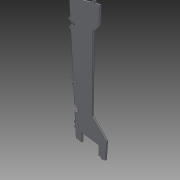
# Autodesk Inventor part: inner_brace_left
Saved by Autodesk Inventor 2014 (Build 180170000, 170)
## iProperties
Created: 2014-04-02
Part Number: inner_brace_left
Material: Plywood, Finish
Document SubType Name: Modeling
Designer: buben
Density: 0.552 g/cm^3
Appearance: Plywood - New
Author: buben
Autodesk Inventor part; units mm, degrees
ref_plane "YZ Plane" through (0, 0, 0) normal (1, 0, 0) x (0, 1, 0)
ref_plane "XZ Plane" through (0, 0, 0) normal (0, 1, 0) x (-1, 0, 0)
ref_plane "XY Plane" through (0, 0, 0) normal (0, 0, 1) x (1, 0, 0)
sketch "Sketch1" plane through (0, 0, 0) normal (0, 1, 0) x (-1, 0, 0)
  line L0 (0, 0) -> (0, -489)
  line L1 (0, -489) -> (-30.25, -489)
  line L2 (-30.25, -489) -> (-30.25, -439)
  line L3 (-30.25, -439) -> (-112.25, -439)
  line L4 (-112.25, -439) -> (-112.25, -489)
  line L5 (-112.25, -489) -> (-142.5, -489)
  line L6 (-142.5, -489) -> (-142.5, -399)
  line L7 (-142.5, -399) -> (-80, -336.5)
  line L8 (-80, -336.5) -> (-80, -65)
  line L9 (-80, -65) -> (-100, -45)
  line L10 (-100, -45) -> (-100, 0)
  line L11 (-100, 0) -> (0, 0)
  dimension "d0" = 135
  dimension "d1" = 100
  dimension "d2" = 489
  dimension "d3" = 45
  dimension "d4" = 20
  dimension "d5" = 30.25
  dimension "d6" = 50
  dimension "d7" = 82
  dimension "d8" = 40
  constraints: 24 end point, 7 parallel, 3 collinear, 2 perpendicular, 1 vertical
  measures "d0" angle of L9 L10
  measures "d1" distance of L10.end L0.start
  measures "d2" distance of L0.start L0.end
  measures "d3" distance of L9.end L10.end
  measures "d4" horizontal distance of L8.end L9.end
  measures "d5" distance of L0.end L1.end
  measures "d6" distance of L1.end L2.end
  measures "d7" distance of L2.end L3.end
  measures "d8" vertical distance of L6.end L3.end
extrude "Extrusion1" add sketch "Sketch1" along normal blind 6.5
sketch "Sketch2" plane through (0, 6.5, 0) normal (0, 1, 0) x (1, 0, 0)
  line L0 (0, 0) -> (100, 0) projected
  line L1 (30.25, 489) -> (0, 489) projected
  line L2 (0, 489) -> (0, 0) projected
  line L3 (16.3, 425.75) -> (16.3, 421.25)
  line L4 (0, 421.25) -> (0, 425.75)
  line L5 (5, 428.25) -> (12.3, 428.25)
  line L6 (12.3, 418.75) -> (5, 418.75)
  line L7 (0, 425.75) -> (5, 425.75)
  line L8 (12.3, 425.75) -> (16.3, 425.75)
  line L9 (16.3, 421.25) -> (12.3, 421.25)
  line L10 (5, 421.25) -> (0, 421.25)
  line L11 (5, 418.75) -> (5, 421.25)
  line L12 (5, 425.75) -> (5, 428.25)
  line L13 (12.3, 428.25) -> (12.3, 425.75)
  line L14 (12.3, 421.25) -> (12.3, 418.75)
  line L15 (16.3, 246.75) -> (16.3, 242.25)
  line L16 (0, 242.25) -> (0, 246.75)
  line L17 (5, 249.25) -> (12.3, 249.25)
  line L18 (12.3, 239.75) -> (5, 239.75)
  line L19 (0, 246.75) -> (5, 246.75)
  line L20 (12.3, 246.75) -> (16.3, 246.75)
  line L21 (16.3, 242.25) -> (12.3, 242.25)
  line L22 (5, 242.25) -> (0, 242.25)
  line L23 (5, 239.75) -> (5, 242.25)
  line L24 (5, 246.75) -> (5, 249.25)
  line L25 (12.3, 249.25) -> (12.3, 246.75)
  line L26 (12.3, 242.25) -> (12.3, 239.75)
  line L27 (16.3, 67.75) -> (16.3, 63.25)
  line L28 (0, 63.25) -> (0, 67.75)
  line L29 (5, 70.25) -> (12.3, 70.25)
  line L30 (12.3, 60.75) -> (5, 60.75)
  line L31 (0, 67.75) -> (5, 67.75)
  line L32 (12.3, 67.75) -> (16.3, 67.75)
  line L33 (16.3, 63.25) -> (12.3, 63.25)
  line L34 (5, 63.25) -> (0, 63.25)
  line L35 (5, 60.75) -> (5, 63.25)
  line L36 (5, 67.75) -> (5, 70.25)
  line L37 (12.3, 70.25) -> (12.3, 67.75)
  line L38 (12.3, 63.25) -> (12.3, 60.75)
  line L39 (8.65, 418.75) -> (8.65, 249.25) construction
  line L40 (8.65, 239.75) -> (8.65, 70.25) construction
  point P0 (16.3, 423.5)
  point P1 (16.3, 244.5)
  point P2 (16.3, 65.5)
  dimension "d11" = 4.5
  dimension "d12" = 5
  dimension "d13" = 4
  dimension "d14" = 7.3
  dimension "d15" = 2.5
  dimension "d16" = 4.5
  dimension "d17" = 5
  dimension "d18" = 4
  dimension "d19" = 7.3
  dimension "d20" = 2.5
  dimension "d21" = 4.5
  dimension "d22" = 5
  dimension "d23" = 4
  dimension "d24" = 7.3
  dimension "d25" = 2.5
  dimension "d26" = 65.5
  dimension "d27" = 65.5
  constraints: 76 end point, 30 parallel, 19 collinear, 12 perpendicular, 9 horizontal, 7 midpoint
  measures "d11" distance of L3.start L3.end
  measures "d12" distance of L10.start L4.start
  measures "d13" distance of L3.end L9.end
  measures "d14" distance of L6.start L6.end
  measures "d15" distance of L5.end L8.start
  measures "d16" distance of L20.end L15.end
  measures "d17" distance of L23.end L16.start
  measures "d18" distance of L15.end L26.start
  measures "d19" distance of L26.end L23.start
  measures "d20" distance of L17.end L20.start
  measures "d21" distance of L32.end L27.end
  measures "d22" distance of L35.end L28.start
  measures "d23" distance of L27.end L38.start
  measures "d24" distance of L38.end L35.start
  measures "d25" distance of L29.end L32.start
  measures "d26" distance from line of L1 point (16.3, 423.5)
  measures "d27" distance from line of L0 point (16.3, 65.5)
extrude "Extrusion2" cut sketch "Sketch2" against normal through all
sketch "Sketch3" plane through (0, 6.5, 0) normal (0, 1, 0) x (1, 0, 0)
  line L0 (0, 242.25) -> (0, 67.75) projected
  line L1 (16.3, 67.75) -> (16.3, 63.25) projected
  line L2 (0, 63.25) -> (0, 0) projected
  line L3 (0, 489) -> (0, 425.75) projected
  line L4 (16.3, 425.75) -> (16.3, 421.25) projected
  line L5 (0, 421.25) -> (0, 246.75) projected
  line L6 (16.3, 246.75) -> (16.3, 242.25) projected
  line L7 (0, 439) -> (-4.5, 439)
  line L8 (-6.5, 437) -> (-6.5, 433)
  line L9 (-4.5, 431) -> (0, 431)
  line L10 (0, 431) -> (0, 439)
  line L11 (0, 416) -> (-4.5, 416)
  line L12 (-6.5, 414) -> (-6.5, 410)
  line L13 (-4.5, 408) -> (0, 408)
  line L14 (0, 408) -> (0, 416)
  line L15 (0, 260) -> (-4.5, 260)
  line L16 (-6.5, 258) -> (-6.5, 254)
  line L17 (-4.5, 252) -> (0, 252)
  line L18 (0, 252) -> (0, 260)
  line L19 (0, 237) -> (-4.5, 237)
  line L20 (-6.5, 235) -> (-6.5, 231)
  line L21 (-4.5, 229) -> (0, 229)
  line L22 (0, 229) -> (0, 237)
  line L23 (0, 81) -> (-4.5, 81)
  line L24 (-6.5, 79) -> (-6.5, 75)
  line L25 (-4.5, 73) -> (0, 73)
  line L26 (0, 73) -> (0, 81)
  line L27 (0, 58) -> (-4.5, 58)
  line L28 (-6.5, 56) -> (-6.5, 52)
  line L29 (-4.5, 50) -> (0, 50)
  line L30 (0, 50) -> (0, 58)
  arc A0 (-4.5, 439) -> (-6.5, 437) centre (-4.5, 437) ccw
  arc A1 (-6.5, 433) -> (-4.5, 431) centre (-4.5, 433) ccw
  arc A2 (-4.5, 416) -> (-6.5, 414) centre (-4.5, 414) ccw
  arc A3 (-6.5, 410) -> (-4.5, 408) centre (-4.5, 410) ccw
  arc A4 (-4.5, 260) -> (-6.5, 258) centre (-4.5, 258) ccw
  arc A5 (-6.5, 254) -> (-4.5, 252) centre (-4.5, 254) ccw
  arc A6 (-4.5, 237) -> (-6.5, 235) centre (-4.5, 235) ccw
  arc A7 (-6.5, 231) -> (-4.5, 229) centre (-4.5, 231) ccw
  arc A8 (-4.5, 81) -> (-6.5, 79) centre (-4.5, 79) ccw
  arc A9 (-6.5, 75) -> (-4.5, 73) centre (-4.5, 75) ccw
  arc A10 (-4.5, 58) -> (-6.5, 56) centre (-4.5, 56) ccw
  arc A11 (-6.5, 52) -> (-4.5, 50) centre (-4.5, 52) ccw
  point P0 (16.3, 423.5)
  point P1 (16.3, 244.5)
  point P2 (16.3, 65.5)
  dimension "d30" = 2
  dimension "d31" = 8
  dimension "d32" = 8
  dimension "d33" = 15
  dimension "d34" = 8
  dimension "d35" = 8
  dimension "d36" = 15
  dimension "d37" = 8
  dimension "d38" = 8
  dimension "d39" = 15
  dimension "d40" = 7.5
  dimension "d41" = 7.5
  dimension "d42" = 7.5
  dimension "d43" = 6.5
  constraints: 48 end point, 24 point on circle, 24 tangent, 12 centre point, 12 parallel, 11 equal radius, 6 horizontal, 6 perpendicular, 6 point on line, 5 collinear, 3 midpoint
  measures "d30" radius of A0
  measures "d31" distance between parallel lines of L9 L7
  measures "d32" distance between parallel lines of L13 L11
  measures "d33" distance between parallel lines of L11 L9
  measures "d34" distance between parallel lines of L17 L15
  measures "d35" distance between parallel lines of L21 L19
  measures "d36" distance between parallel lines of L19 L17
  measures "d37" distance between parallel lines of L25 L23
  measures "d38" distance between parallel lines of L27 L29
  measures "d39" distance between parallel lines of L27 L25
  measures "d40" distance from line of point (16.3, 65.5) L25
  measures "d41" distance from line of point (16.3, 244.5) L17
  measures "d42" distance from line of point (16.3, 423.5) L9
  measures "d43" distance between parallel lines of L3 L8
extrude "Extrusion3" add sketch "Sketch3" against normal blind 6.5
sketch "Sketch4" plane through (0, 6.5, 0) normal (0, 1, 0) x (1, 0, 0)
  line L0 (0, 0) -> (100, 0) projected
  line L1 (100, 0) -> (100, 45) projected
  line L2 (142.5, 399) -> (142.5, 489) projected
  line L3 (142.5, 489) -> (112.25, 489) projected
  line L4 (77, 0) -> (85, 0)
  line L5 (85, 0) -> (85, -4.5)
  line L6 (83, -6.5) -> (79, -6.5)
  line L7 (77, -4.5) -> (77, 0)
  line L8 (124.5, 489) -> (132.5, 489)
  line L9 (132.5, 489) -> (132.5, 493.5)
  line L10 (130.5, 495.5) -> (126.5, 495.5)
  line L11 (124.5, 493.5) -> (124.5, 489)
  arc A0 (126.5, 495.5) -> (124.5, 493.5) centre (126.5, 493.5) ccw
  arc A1 (132.5, 493.5) -> (130.5, 495.5) centre (130.5, 493.5) ccw
  arc A2 (83, -6.5) -> (85, -4.5) centre (83, -4.5) ccw
  arc A3 (77, -4.5) -> (79, -6.5) centre (79, -4.5) ccw
  dimension "d46" = 2
  dimension "d47" = 8
  dimension "d48" = 6.5
  dimension "d49" = 15
  dimension "d50" = 8
  dimension "d51" = 6.5
  dimension "d52" = 10
  constraints: 16 end point, 8 point on circle, 8 tangent, 4 centre point, 4 parallel, 3 equal radius, 2 horizontal, 2 perpendicular, 2 point on line
  measures "d46" radius of A0
  measures "d47" distance between parallel lines of L5 L7
  measures "d48" distance between parallel lines of L0 L6
  measures "d49" distance between parallel lines of L1 L5
  measures "d50" distance between parallel lines of L9 L11
  measures "d51" distance between parallel lines of L3 L10
  measures "d52" distance between parallel lines of L2 L9
extrude "Extrusion4" add sketch "Sketch4" against normal blind 6.5
sketch "Sketch5" plane through (0, 6.5, 0) normal (0, 1, 0) x (1, 0, 0)
  line L0 (30.25, 489) -> (0, 489) projected
  line L1 (0, 408) -> (0, 260) projected
  line L2 (8.6603, 332.75) -> (0, 332.75)
  line L3 (0, 362.75) -> (8.6603, 362.75)
  line L4 (8.6603, 362.75) -> (17.3205, 347.75)
  line L5 (17.3205, 347.75) -> (8.6603, 332.75)
  line L6 (0, 362.75) -> (0, 332.75)
  point P0 (0, 347.75)
  dimension "d55" = 30
  dimension "d56" = 156.25
  constraints: 10 end point, 3 point on line, 1 collinear, 1 horizontal, 1 parallel, 6 other
  measures "d55" distance between parallel lines of L2 L3
  measures "d56" distance between parallel lines of L2 L0
extrude "Extrusion5" cut sketch "Sketch5" against normal through all
chamfer "Chamfer1" distance 4 angle 45 1 edges at (0, 3.25, 0)
equation "\"d27\" = d26"
equation "\"d32\" = d31"
equation "\"d34\" = d32"
equation "\"d35\" = d34"
equation "\"d36\" = d33"
equation "\"d37\" = d35"
equation "\"d38\" = d37"
equation "\"d39\" = d36"
equation "\"d40\" = 0.5 * d39"
equation "\"d41\" = d40"
equation "\"d42\" = d41"
equation "\"d50\" = d47"
equation "\"d51\" = d48"
body "Solid1"
